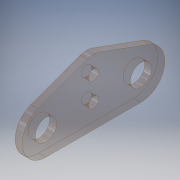
# Autodesk Inventor part: Bottom Roler Bearing Holder
Saved by Autodesk Inventor 2019.4 (Build 234330000, 330)
## iProperties
Created: 2020-01-11
Part Number: Bottom Roler Bearing Holder
Material: Polycarbonate, Smoke
Document SubType Name: Modeling
Designer: admin
Density: 1.2 g/cm^3
Appearance: Polycarbonate - Smoked
Author: admin
Autodesk Inventor part; units mm, degrees
ref_plane "YZ Plane" through (0, 0, 0) normal (1, 0, 0) x (0, 1, 0)
ref_plane "XZ Plane" through (0, 0, 0) normal (0, 1, 0) x (-1, 0, 0)
ref_plane "XY Plane" through (0, 0, 0) normal (0, 0, 1) x (1, 0, 0)
sketch "Sketch1" plane through (0, 0, 0) normal (1, 0, 0) x (0, 1, 0)
  circle A0 centre (0, 20) radius 4.5
  circle A1 centre (0, -20) radius 4.5
  line L0 (0, -20) -> (0, 20) construction
  circle A2 centre (0, 0) radius 2.2
  circle A3 centre (10, 0) radius 2.2
  line L1 (0, 0) -> (10, 0) construction
  arc A4 (-10, 20) -> (9.3882, 23.4441) centre (0, 20) ccw construction
  arc A5 (9.3882, -23.4441) -> (-10, -20) centre (0, -20) ccw construction
  arc A6 (17.0411, 2.5831) -> (17.0411, -2.5831) centre (10, 0) ccw construction
  line L2 (9.3882, -23.4441) -> (17.0411, -2.5831)
  line L3 (17.0411, 2.5831) -> (9.3882, 23.4441)
  line L4 (-10, 20) -> (-10, -20)
  arc A7 (9.3882, 23.4441) -> (-10, 20) centre (0, 20) ccw
  arc A8 (-10, -20) -> (9.3882, -23.4441) centre (0, -20) ccw
  arc A9 (17.0411, -2.5831) -> (17.0411, 2.5831) centre (10, 0) ccw
  dimension "d0" = 9
  dimension "d1" = 9
  dimension "d2" = 40
  dimension "d3" = 4.4
  dimension "d4" = 4.4
  dimension "d5" = 10
  dimension "d6" = 20
  dimension "d7" = 20
  dimension "d8" = 15
  constraints: 12 point on circle, 10 centre point, 10 end point, 6 tangent, 5 coincident, 1 horizontal, 1 midpoint, 1 vertical
  measures "d0" diameter of A0
  measures "d1" diameter of A1
  measures "d2" distance of L0.start L0.end
  measures "d3" diameter of A2
  measures "d4" diameter of A3
  measures "d5" distance of L1.start L1.end
  measures "d6" diameter of A4
  measures "d7" diameter of A5
  measures "d8" diameter of A6
extrude "Extrusion1" add sketch "Sketch1" along normal blind 3
body "Solid1"
